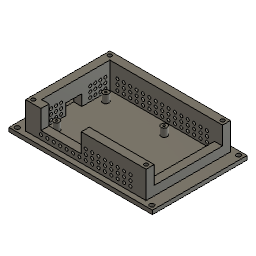
RPi+Board+Case (Autodesk Fusion 360 design; units mm, degrees)
Autodesk Fusion 360 part; units mm, degrees
note: some values were not read from the file. Set by a fixed rule: which sketch regions a step uses.
sketch "Sketch1" plane through (0, 0, 0) normal (0, 1, 0) x (1, 0, 0)
  line L0 (-60, 42) -> (60, 42)
  line L1 (60, 42) -> (60, -42)
  line L2 (60, -42) -> (-60, -42)
  line L3 (-60, -42) -> (-60, 42)
  dimension "d1" = 120
  dimension "d2" = 84
  dimension "d3" = 60
  dimension "d4" = 42
  constraint horizontal L0
  constraint vertical L1
  constraint horizontal L2
  constraint vertical L3
  measures "d1" distance of L0.start L0.end
  measures "d2" distance of L0.start L2.end
  measures "d3" distance of origin L1
  measures "d4" distance of origin L0
extrude "Extrude1" add sketch "Sketch1" along normal blind 5 makes body 1
sketch "Sketch2" plane through (0, 5, 0) normal (0, 1, 0) x (-1, 0, 0)
  line L0 (60, 42) -> (-60, 42)
  line L1 (-60, 42) -> (-60, -42)
  line L2 (-60, -42) -> (60, -42)
  line L3 (60, -42) -> (60, 42)
  line L4 (52, -34) -> (-52, -34)
  line L5 (-52, -34) -> (-52, 34)
  line L6 (-52, 34) -> (52, 34)
  line L7 (52, 34) -> (52, -34)
  dimension "d7" = 8
  dimension "d8" = 8
  dimension "d9" = 8
  dimension "d10" = 8
  constraint horizontal L4
  constraint vertical L5
  constraint horizontal L6
  constraint vertical L7
  measures "d7" distance of L3 L7
  measures "d8" distance of L2 L4
  measures "d9" distance of L1 L5
  measures "d10" distance of L0 L6
extrude "Extrude2" add sketch "Sketch2" along normal blind 26 bodies 1
sketch "Sketch3" plane through (0, 5, 0) normal (0, 1, 0) x (-1, 0, 0)
  line L0 (-52, 34) -> (-52, -34)
  line L1 (-52, -34) -> (52, -34)
  line L2 (52, -34) -> (52, 34)
  line L3 (52, 34) -> (-52, 34)
  line L4 (44.5, -22.5) -> (-13.5, -22.5) construction
  line L5 (-13.5, -22.5) -> (-13.5, 26.5) construction
  line L6 (-13.5, 26.5) -> (44.5, 26.5) construction
  line L7 (44.5, 26.5) -> (44.5, -22.5) construction
  circle A0 centre (44.5, -22.5) radius 1.05
  circle A1 centre (-13.5, -22.5) radius 1.05
  circle A2 centre (-13.5, 26.5) radius 1.05
  circle A3 centre (44.5, 26.5) radius 1.05
  circle A4 centre (44.5, -22.5) radius 3.05
  circle A5 centre (-13.5, -22.5) radius 3.05
  circle A6 centre (-13.5, 26.5) radius 3.05
  circle A7 centre (44.5, 26.5) radius 3.05
  dimension "d13" = 58
  dimension "d14" = 49
  dimension "d15" = 11.5
  dimension "d16" = 7.5
  dimension "d17" = 2.1
  dimension "d18" = 2.1
  dimension "d19" = 2.1
  dimension "d20" = 2.1
  dimension "d21" = 6.1
  dimension "d22" = 6.1
  dimension "d23" = 6.1
  dimension "d24" = 6.1
  dimension "d50" = 38.5
  constraint horizontal L4
  constraint vertical L5
  constraint horizontal L6
  constraint vertical L7
  constraint coincident L4.start L7.end
  constraint coincident L4.end L5.start
  constraint coincident L5.end L6.start
  constraint coincident L6.end L7.start
  constraint concentric A0 A4
  constraint concentric A1 A5
  constraint concentric A2 A6
  constraint concentric A3 A7
  measures "d13" distance of L4.start L4.end
  measures "d14" distance of L4.start L6.end
  measures "d15" distance of L1 L4
  measures "d16" distance of L2 L7
  measures "d17" diameter of A0
  measures "d18" diameter of A1
  measures "d19" diameter of A2
  measures "d20" diameter of A3
  measures "d21" diameter of A4
  measures "d22" diameter of A5
  measures "d23" diameter of A6
  measures "d24" diameter of A7
  measures "d50" distance of L0 L5
extrude "Extrude3" add sketch "Sketch3" along normal blind 8 contours A4 | A5 | A6 | A7 bodies 1
sketch "Sketch4" plane through (0, 0, 42) normal (0, 0, 1) x (1, 0, 0)
  line L0 (-60, 0) -> (60, 0)
  line L1 (60, 0) -> (60, 31)
  line L2 (60, 31) -> (-60, 31)
  line L3 (-60, 31) -> (-60, 0)
  line L4 (-47.55, 5) -> (-41.45, 5)
  line L5 (10.45, 5) -> (16.55, 5)
  line L6 (52, 5) -> (-52, 5)
  line L7 (-52, 5) -> (52, 5)
  line L8 (10.45, 5) -> (16.55, 5)
  line L9 (-47.55, 5) -> (-41.45, 5)
  line L10 (-44.5, 32) -> (-4.5, 32)
  line L11 (-4.5, 32) -> (-4.5, 12)
  line L12 (-4.5, 12) -> (-44.5, 12)
  line L13 (-44.5, 12) -> (-44.5, 32)
  line L14 (-44.5, 12) -> (-44.5, 5) construction
  circle A0 centre (-44.5, 8.5) radius 1.5
  circle A1 centre (-38.1429, 8.5) radius 1.5
  circle A2 centre (-31.7857, 8.5) radius 1.5
  circle A3 centre (-25.4286, 8.5) radius 1.5
  circle A4 centre (-19.0714, 8.5) radius 1.5
  circle A5 centre (-12.7143, 8.5) radius 1.5
  circle A6 centre (-6.3571, 8.5) radius 1.5
  circle A7 centre (0, 8.5) radius 1.5
  circle A8 centre (6.3571, 8.5) radius 1.5
  circle A9 centre (12.7143, 8.5) radius 1.5
  circle A10 centre (19.0714, 8.5) radius 1.5
  circle A11 centre (25.4286, 8.5) radius 1.5
  circle A12 centre (31.7857, 8.5) radius 1.5
  circle A13 centre (38.1429, 8.5) radius 1.5
  circle A14 centre (44.5, 8.5) radius 1.5
  circle A15 centre (12.7143, 13.5) radius 1.5
  circle A16 centre (6.3571, 13.5) radius 1.5
  circle A17 centre (38.1429, 13.5) radius 1.5
  circle A18 centre (25.4286, 13.5) radius 1.5
  circle A19 centre (44.5, 13.5) radius 1.5
  circle A20 centre (0, 13.5) radius 1.5
  circle A21 centre (19.0714, 13.5) radius 1.5
  circle A22 centre (31.7857, 13.5) radius 1.5
  circle A23 centre (12.7143, 18.5) radius 1.5
  circle A24 centre (6.3571, 18.5) radius 1.5
  circle A25 centre (38.1429, 18.5) radius 1.5
  circle A26 centre (25.4286, 18.5) radius 1.5
  circle A27 centre (44.5, 18.5) radius 1.5
  circle A28 centre (0, 18.5) radius 1.5
  circle A29 centre (19.0714, 18.5) radius 1.5
  circle A30 centre (31.7857, 18.5) radius 1.5
  point P0 (-44.5, 8.5)
  dimension "d27" = 7
  dimension "d29" = 40
  dimension "d38" = 1
  dimension "d74" = 3
  dimension "d77" = 89
  dimension "d78" = 5
  dimension "d79" = 7.5
  dimension "d80" = 7.5
  dimension "d102" = 0
  dimension "d103" = 10
  constraint horizontal L10
  constraint vertical L11
  constraint horizontal L12
  constraint vertical L13
  constraint midpoint L4 L14.end
  constraint perpendicular L6 L14
  constraint midpoint L14 P0
  constraint coincident P0 A0.centre
  measures "d27" distance of L6 L12
  measures "d29" distance of L10.start L10.end
  measures "d38" distance of L2 L10
  measures "d74" diameter of A0
  measures "d79" horizontal distance of L6.end P0
  measures "d80" horizontal distance of L6.start A14.centre
extrude "Extrude4" cut sketch "Sketch4" against normal up to surface (8 mm away) contours L2 L10 L11 L13 | L2 L11 L12 L13 | A0 | A1 | A2 | A3 | A4 | A5 | A6 | A7 | A8 | A9 | A10 | A11 | A12 | A13 | A14 | A15 | A16 | A17 | A18 | A19 | A20 | A21 | A22 | A23 | A24 | A25 | A26 | A27 | A28 | A29 | A30 bodies 1
sketch "Sketch5" plane through (60, 0, 0) normal (1, 0, 0) x (0, 0, -1)
  line L0 (-42, 0) -> (42, 0)
  line L1 (42, 0) -> (42, 31)
  line L2 (42, 31) -> (-42, 31)
  line L3 (-42, 31) -> (-42, 0)
  line L4 (19.45, 5) -> (25.55, 5)
  line L5 (19.45, 5) -> (25.55, 5)
  line L6 (-34, 5) -> (34, 5)
  line L7 (34, 5) -> (-34, 5)
  line L8 (-29.55, 5) -> (-23.45, 5)
  line L9 (-29.55, 5) -> (-23.45, 5)
  line L10 (-34, 31) -> (34, 31)
  line L11 (34, 31) -> (34, 13)
  line L12 (34, 13) -> (-34, 13)
  line L13 (-34, 13) -> (-34, 31)
  point P0 (-34, 31)
  point P1 (34, 31)
  dimension "d34" = 8
  constraint horizontal L10
  constraint vertical L11
  constraint horizontal L12
  constraint vertical L13
  constraint coincident L2 P0
  constraint coincident L13 P0
  constraint coincident L11 P1
  measures "d34" distance of L7 L12
extrude "Extrude5" cut sketch "Sketch5" against normal up to surface (8 mm away) contours L2 L10 L11 L12 L13 bodies 1
sketch "Sketch6" plane through (0, 31, 0) normal (0, 1, 0) x (-1, 0, 0)
  line L0 (-60, -34) -> (-60, -42)
  line L1 (-60, -42) -> (60, -42)
  line L2 (60, -42) -> (60, 42)
  line L3 (60, 42) -> (44.5, 42)
  line L4 (44.5, 42) -> (44.5, 34)
  line L5 (44.5, 34) -> (52, 34)
  line L6 (52, 34) -> (52, -34)
  line L7 (52, -34) -> (-60, -34)
  line L8 (-60, -34) -> (-60, -42) construction
  line L9 (-60, -34) -> (-60, -32) construction
  line L10 (-60, 34) -> (4.5, 34) construction
  line L11 (4.5, 34) -> (4.5, 42) construction
  line L12 (4.5, 42) -> (-60, 42) construction
  line L13 (-60, 42) -> (-60, 34) construction
  circle A0 centre (56, -38) radius 1.9
  circle A1 centre (-56, -38) radius 1.9
  circle A2 centre (-56, 38) radius 1.9
  circle A3 centre (56, 38) radius 1.9
  line L14 (-56, 38) -> (56, 38) construction
  line L15 (56, 38) -> (56, -38) construction
  line L16 (56, -38) -> (-56, -38) construction
  line L17 (-56, -38) -> (-56, 38) construction
  line L18 (-52, -34) -> (-52, 34) construction
  line L19 (-52, 34) -> (-60, 34) construction
  line L20 (-60, 34) -> (-60, -34) construction
  line L21 (-60, -34) -> (-52, -34) construction
  line L22 (52, -34) -> (60, -34) construction
  line L23 (52, -34) -> (52, -42) construction
  point P0 (-56, -34)
  point P1 (4.5, 38)
  point P2 (56, -34)
  point P3 (52, -38)
  dimension "d39" = 3.8
  dimension "d40" = 3.8
  dimension "d41" = 3.8
  dimension "d42" = 3.8
  constraint coincident L0.start L7.end
  constraint coincident L1 L0.end
  constraint perpendicular L1 L8
  constraint coincident L0 L9.end
  constraint coincident A2.centre L14.start
  constraint coincident A3.centre L14.end
  constraint parallel L3 L14
  constraint coincident A0.centre L15.end
  constraint coincident A1.centre L16.end
  constraint perpendicular L15 L16
  constraint perpendicular L14 L17
  constraint perpendicular L14 L15
  constraint midpoint L21 P0
  constraint coincident L17 P0
  constraint midpoint L11 P1
  constraint coincident L14 P1
  constraint coincident L6.end L7.start
  constraint coincident L2 L22.end
  constraint perpendicular L2 L22
  constraint coincident L1 L23.end
  constraint perpendicular L1 L23
  constraint midpoint L22 P2
  constraint midpoint L23 P3
  constraint coincident L16 P3
  constraint coincident L15 P2
  measures "d39" diameter of A0
  measures "d40" diameter of A1
  measures "d41" diameter of A2
  measures "d42" diameter of A3
extrude "Extrude6" cut sketch "Sketch6" against normal blind 10 contours A0 | A1 | A2 | A3 bodies 1
sketch "Sketch7" plane through (-60, 0, 0) normal (-1, 0, 0) x (0, 0, 1)
  line L0 (-42, 0) -> (42, 0)
  line L1 (42, 0) -> (42, 31)
  line L2 (42, 31) -> (-42, 31)
  line L3 (-42, 31) -> (-42, 0)
  line L4 (-19.45, 13) -> (-25.55, 13)
  line L5 (29.55, 13) -> (23.45, 13)
  line L6 (-25.55, 13) -> (29.55, 13) construction
  line L7 (-25.55, 5) -> (-19.45, 5)
  line L8 (-25.55, 5) -> (-19.45, 5)
  line L9 (34, 5) -> (-34, 5)
  line L10 (-34, 5) -> (34, 5)
  line L11 (23.45, 5) -> (29.55, 5)
  line L12 (23.45, 5) -> (29.55, 5)
  line L13 (-6, 16) -> (10, 16)
  line L14 (10, 16) -> (10, 5)
  line L15 (10, 5) -> (-6, 5)
  line L16 (-6, 5) -> (-6, 16)
  line L17 (2, 16) -> (2, 13) construction
  line L18 (-23.55, 13) -> (-21.45, 13)
  line L19 (25.45, 13) -> (27.55, 13)
  point P0 (2, 13)
  point P1 (2, 16)
  point P2 (0, 5)
  dimension "d54" = 16
  dimension "d55" = 3
  constraint coincident L4.end L6.start
  constraint coincident L5.start L6.end
  constraint midpoint L6 P0
  constraint horizontal L13
  constraint vertical L14
  constraint horizontal L15
  constraint vertical L16
  constraint midpoint L13 P1
  constraint coincident P1 L17.start
  constraint coincident P0 L17.end
  constraint vertical L17
  constraint midpoint L10 P2
  constraint coincident L15 P2
  measures "d54" distance of L13.start L13.end
  measures "d55" distance of P1 P0
extrude "Extrude7" cut sketch "Sketch7" against normal up to surface (8 mm away) contours L9 L10 L13 L14 L15 L16 bodies 1
sketch "Sketch8" plane through (0, 0, 0) normal (0, -1, 0) x (1, 0, 0)
  line L0 (-60, -42) -> (60, -42)
  line L1 (60, -42) -> (60, 42)
  line L2 (60, 42) -> (-60, 42)
  line L3 (-60, 42) -> (-60, -42)
  line L4 (-71.4, 47.15) -> (71.4, 47.15)
  line L5 (71.4, 47.15) -> (71.4, -47.15)
  line L6 (71.4, -47.15) -> (-71.4, -47.15)
  line L7 (-71.4, -47.15) -> (-71.4, 47.15)
  circle A0 centre (-66.9, -43.15) radius 2.25
  circle A1 centre (66.9, -43.15) radius 2.25
  circle A2 centre (66.9, 43.15) radius 2.25
  circle A3 centre (-66.9, 43.15) radius 2.25
  line L8 (-66.9, -43.15) -> (66.9, -43.15) construction
  line L9 (66.9, -43.15) -> (66.9, 43.15) construction
  line L10 (66.9, 43.15) -> (-66.9, 43.15) construction
  line L11 (-66.9, 43.15) -> (-66.9, -43.15) construction
  dimension "d60" = 142.8
  dimension "d61" = 94.3
  dimension "d62" = 71.4
  dimension "d63" = 47.15
  dimension "d64" = 4.5
  dimension "d65" = 4
  dimension "d66" = 4.5
  dimension "d67" = 4.5
  dimension "d68" = 4.5
  dimension "d69" = 4.5
  dimension "d70" = 4.5
  dimension "d71" = 4
  constraint horizontal L4
  constraint vertical L5
  constraint horizontal L6
  constraint vertical L7
  constraint coincident A0.centre L8.start
  constraint coincident A1.centre L8.end
  constraint coincident A2.centre L9.end
  constraint coincident A3.centre L10.end
  constraint horizontal L10
  constraint perpendicular L8 L11
  constraint perpendicular L8 L9
  constraint perpendicular L9 L10
  measures "d60" distance of L4.start L4.end
  measures "d61" distance of L4.start L6.end
  measures "d62" distance of origin L5
  measures "d63" distance of origin L4
  measures "d64" distance of L7 A0.centre
  measures "d65" distance of L6 A0.centre
  measures "d66" distance of L5 A1.centre
  measures "d67" diameter of A0
  measures "d68" diameter of A1
  measures "d69" diameter of A3
  measures "d70" diameter of A2
  measures "d71" distance of L4 A3.centre
extrude "Extrude8" add sketch "Sketch8" against normal blind 4 separate body makes body 2
sketch "Sketch10" plane through (0, 0, -42) normal (0, 0, -1) x (-1, 0, 0)
  line L0 (60, 31) -> (-60, 31)
  line L1 (-60, 0) -> (60, 0)
  circle A0 centre (-44.5, 8.5) radius 1.5
  circle A1 centre (-38.1429, 8.5) radius 1.5
  circle A2 centre (-31.7857, 8.5) radius 1.5
  circle A3 centre (-25.4286, 8.5) radius 1.5
  circle A4 centre (-19.0714, 8.5) radius 1.5
  circle A5 centre (-12.7143, 8.5) radius 1.5
  circle A6 centre (-6.3571, 8.5) radius 1.5
  circle A7 centre (0, 8.5) radius 1.5
  circle A8 centre (6.3571, 8.5) radius 1.5
  circle A9 centre (12.7143, 8.5) radius 1.5
  circle A10 centre (19.0714, 8.5) radius 1.5
  circle A11 centre (25.4286, 8.5) radius 1.5
  circle A12 centre (31.7857, 8.5) radius 1.5
  circle A13 centre (38.1429, 8.5) radius 1.5
  circle A14 centre (44.5, 8.5) radius 1.5
  circle A15 centre (25.4286, 13.5) radius 1.5
  circle A16 centre (6.3571, 13.5) radius 1.5
  circle A17 centre (44.5, 13.5) radius 1.5
  circle A18 centre (31.7857, 13.5) radius 1.5
  circle A19 centre (-31.7857, 13.5) radius 1.5
  circle A20 centre (19.0714, 13.5) radius 1.5
  circle A21 centre (38.1429, 13.5) radius 1.5
  circle A22 centre (0, 13.5) radius 1.5
  circle A23 centre (-19.0714, 13.5) radius 1.5
  circle A24 centre (12.7143, 13.5) radius 1.5
  circle A25 centre (-25.4286, 13.5) radius 1.5
  circle A26 centre (-12.7143, 13.5) radius 1.5
  circle A27 centre (-6.3571, 13.5) radius 1.5
  circle A28 centre (-38.1429, 13.5) radius 1.5
  circle A29 centre (-44.5, 13.5) radius 1.5
  circle A30 centre (25.4286, 18.5) radius 1.5
  circle A31 centre (6.3571, 18.5) radius 1.5
  circle A32 centre (44.5, 18.5) radius 1.5
  circle A33 centre (31.7857, 18.5) radius 1.5
  circle A34 centre (-31.7857, 18.5) radius 1.5
  circle A35 centre (19.0714, 18.5) radius 1.5
  circle A36 centre (38.1429, 18.5) radius 1.5
  circle A37 centre (0, 18.5) radius 1.5
  circle A38 centre (-19.0714, 18.5) radius 1.5
  circle A39 centre (12.7143, 18.5) radius 1.5
  circle A40 centre (-25.4286, 18.5) radius 1.5
  circle A41 centre (-12.7143, 18.5) radius 1.5
  circle A42 centre (-6.3571, 18.5) radius 1.5
  circle A43 centre (-38.1429, 18.5) radius 1.5
  circle A44 centre (-44.5, 18.5) radius 1.5
  line L2 (60, 0) -> (60, 31)
  line L3 (-60, 31) -> (-60, 0)
  dimension "d98" = 0
  dimension "d99" = 10
extrude "Extrude9" cut sketch "Sketch10" against normal up to surface (8 mm away) contours A0 | A1 | A2 | A3 | A4 | A5 | A6 | A7 | A8 | A9 | A10 | A11 | A12 | A13 | A14 | A15 | A16 | A17 | A18 | A19 | A20 | A21 | A22 | A23 | A24 | A25 | A26 | A27 | A28 | A29 | A30 | A31 | A32 | A33 | A34 | A35 | A36 | A37 | A38 | A39 | A40 | A41 | A42 | A43 | A44 bodies 1
sketch "Sketch11" plane through (-60, 0, 0) normal (-1, 0, 0) x (0, 0, 1)
  line L0 (-42, 0) -> (42, 0)
  line L1 (42, 31) -> (-42, 31)
  line L2 (-42, 7) -> (-42, 10)
  line L3 (-42, 8.5) -> (41.5, 8.5) construction
  circle A0 centre (-29.5, 8.5) radius 1.5
  circle A1 centre (-24.5, 8.5) radius 1.5
  circle A2 centre (-19.5, 8.5) radius 1.5
  circle A3 centre (-14.5, 8.5) radius 1.5
  circle A4 centre (29.5, 8.5) radius 1.5
  circle A5 centre (24.5, 8.5) radius 1.5
  circle A6 centre (19.5, 8.5) radius 1.5
  circle A7 centre (14.5, 8.5) radius 1.5
  circle A8 centre (-29.5, 13.5) radius 1.5
  circle A9 centre (-24.5, 13.5) radius 1.5
  circle A10 centre (-19.5, 13.5) radius 1.5
  circle A11 centre (-14.5, 13.5) radius 1.5
  circle A12 centre (-29.5, 18.5) radius 1.5
  circle A13 centre (-24.5, 18.5) radius 1.5
  circle A14 centre (-19.5, 18.5) radius 1.5
  circle A15 centre (-14.5, 18.5) radius 1.5
  circle A16 centre (29.5, 13.5) radius 1.5
  circle A17 centre (24.5, 13.5) radius 1.5
  circle A18 centre (19.5, 13.5) radius 1.5
  circle A19 centre (14.5, 13.5) radius 1.5
  circle A20 centre (29.5, 18.5) radius 1.5
  circle A21 centre (24.5, 18.5) radius 1.5
  circle A22 centre (19.5, 18.5) radius 1.5
  circle A23 centre (14.5, 18.5) radius 1.5
  line L4 (-6, 5) -> (-6, 16)
  line L5 (-6, 16) -> (10, 16)
  line L6 (10, 16) -> (10, 5)
  line L7 (10, 5) -> (-6, 5)
  line L8 (42, 0) -> (42, 31)
  line L9 (-42, 31) -> (-42, 0)
  dimension "d84" = 3
  dimension "d87" = 15
  dimension "d88" = 10
  dimension "d91" = -15
  dimension "d92" = 10
  constraint midpoint L2 L3.start
  constraint coincident L3 A0.centre
  constraint coincident L3 A4.centre
  constraint equal A0 A4
  measures "d84" diameter of A0
extrude "Extrude10" cut sketch "Sketch11" against normal up to surface (8 mm away) contours A0 | A1 | A2 | A3 | A4 | A5 | A6 | A7 | A8 | A9 | A10 | A11 | A12 | A13 | A14 | A15 | A16 | A17 | A18 | A19 | A20 | A21 | A22 | A23 bodies 1
fillet "Fillet1" [suppressed]
fillet "Fillet2" [suppressed]
equation "d3 = d1 / 2"
equation "d4 = d2 / 2"
equation "d8 = d7"
equation "d9 = d7"
equation "d10 = d7"
equation "d18 = d17"
equation "d19 = d17"
equation "d20 = d17"
equation "d21 = d17 + 4 mm"
equation "d22 = d21"
equation "d23 = d21"
equation "d24 = d21"
equation "d25 = 8.00 mm"
equation "d27 = d25 - 1 mm"
equation "d32 = 2 mm"
equation "d33 = d32"
equation "d34 = d25"
equation "d40 = d39"
equation "d41 = d39"
equation "d42 = d39"
equation "d62 = d60 / 2"
equation "d63 = d61 / 2"
equation "d66 = d64"
equation "d68 = d67"
equation "d69 = d67"
equation "d70 = d67"
